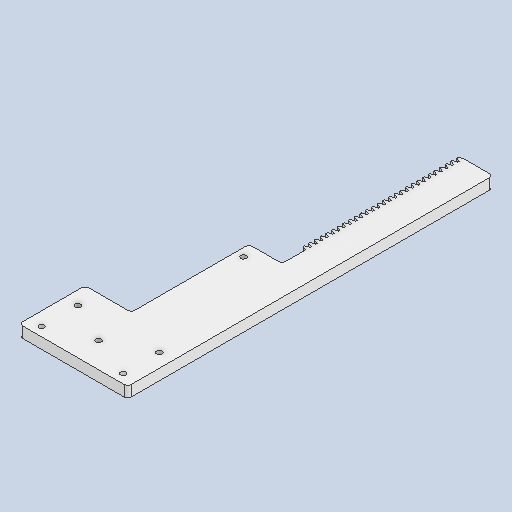
# Autodesk Inventor part: hand-grab-v2-Plate-rack
Saved by Autodesk Inventor 2025.1 (Build 291241000, 241)
## iProperties
Created: 2024-10-12
Part Number: hand-grab-v2-Plate-rack
Material: ABS プラスチック
Document SubType Name: Modeling
Designer: haruy
Density: 1.06 g/cm^3
Appearance: 滑らか - 白
Author: haruy
Autodesk Inventor part; units mm, degrees
ref_plane "YZ Plane" through (0, 0, 0) normal (1, 0, 0) x (0, 1, 0)
ref_plane "XZ Plane" through (0, 0, 0) normal (0, 1, 0) x (-1, 0, 0)
ref_plane "XY Plane" through (0, 0, 0) normal (0, 0, 1) x (1, 0, 0)
derived "hand-grab-v2-Sketch-Base.ipt"
sketch "スケッチ1" plane through (300, 0, 0) normal (1, 0, 0) x (0, 1, 0)
  circle A0 centre (0, 0) radius 122.5
  line L0 (-136.5, 142.5) -> (-132.5, 142.5)
  line L1 (-132.5, 142.5) -> (-132.5, -206.7109)
  line L2 (-132.5, -206.7109) -> (-136.5, -206.7109)
  line L3 (-136.5, -206.7109) -> (-136.5, 142.5)
  line L4 (0, 0) -> (86.6206, 86.6206)
  line L5 (0, 0) -> (0, 122.5)
  line L6 (0, 0) -> (-61.25, 106.0881)
  line L7 (-150.5, 12.2) -> (-198.3, 12.2)
  line L8 (-198.3, 12.2) -> (-198.3, -12.2)
  line L9 (-198.3, -12.2) -> (-150.5, -12.2)
  line L10 (-150.5, -12.2) -> (-150.5, 12.2)
  line L11 (-150.5, 6.5) -> (-147.9, 6.5)
  line L12 (-147.9, 6.5) -> (-147.9, -6.5)
  line L13 (-147.9, -6.5) -> (-150.5, -6.5)
  line L14 (-150.5, -6.5) -> (-150.5, 6.5)
  line L15 (-147.9, 3) -> (-133.5, 3)
  line L16 (-133.5, 3) -> (-133.5, -3)
  line L17 (-133.5, -3) -> (-147.9, -3)
  line L18 (-147.9, -3) -> (-147.9, 3)
  line L19 (-146.5, 70.3296) -> (-150.5, 70.3296)
  line L20 (-150.5, 70.3296) -> (-150.5, -72.1331)
  line L21 (-150.5, -72.1331) -> (-146.5, -72.1331)
  line L22 (-146.5, -72.1331) -> (-146.5, 70.3296)
  line L23 (-136.5, 9) -> (-142.5, 9)
  line L24 (-142.5, 9) -> (-142.5, -9)
  line L25 (-142.5, -9) -> (-136.5, -9)
  line L26 (-136.5, -9) -> (-136.5, 9)
  line L27 (-61.25, 106.0881) -> (-132.5, 106.0881)
  circle A1 centre (-532.5, 0) radius 600
  line L28 (-132.5, 142.5) -> (-7.6064, 142.5)
  arc A2 (86.6206, 86.6206) -> (-7.6064, 142.5) centre (3, 53) ccw
  circle A3 centre (-532.5, 0) radius 400
  circle A4 centre (-332.5, 0) radius 600
sketch "スケッチ2" plane through (0, -300, 0) normal (0, 1, 0) x (-1, 0, 0)
  circle A0 centre (0, 0) radius 122.5
  line L0 (-34, 142.5) -> (-30, 142.5)
  line L1 (-30, 142.5) -> (-30, 106)
  line L2 (-30, 106) -> (-34, 106)
  line L3 (-34, 106) -> (-34, 142.5)
  line L4 (30, 142.5) -> (34, 142.5)
  line L5 (34, 142.5) -> (34, 106)
  line L6 (34, 106) -> (30, 106)
  line L7 (30, 106) -> (30, 142.5)
  circle A1 centre (0, 0) radius 12.5
  line L8 (-30, 142.5) -> (30, 142.5)
  line L9 (-12.5, 103.9737) -> (-12.5, -60) construction
  line L10 (-12.5, -60) -> (-30, -60)
  line L11 (-30, -60) -> (-30, 142.5)
  line L12 (-30, 142.5) -> (-12.5, 142.5)
  line L13 (-12.5, 142.5) -> (-12.5, -60) construction
  line L14 (-30, 20) -> (-12.5, 20) construction
  line L15 (-4.5, 136) -> (4.5, 136) construction
  line L16 (4.5, 136) -> (4.5, 41)
  line L17 (4.5, 41) -> (-4.5, 41) construction
  line L18 (-4.5, 41) -> (-4.5, 136) construction
  line L19 (10, 128.5) -> (-10, 128.5) construction
  line L20 (-10, 128.5) -> (-10, 98.5) construction
  line L21 (-10, 98.5) -> (10, 98.5) construction
  line L22 (10, 98.5) -> (10, 128.5) construction
  line L23 (-12.5, 20) -> (-11.5, 20)
  line L24 (-11.5, 20) -> (-11.5, -60)
  line L25 (-11.5, -60) -> (-12.5, -60)
  line L26 (-12.5, -60) -> (-12.5, 20) construction
  line L27 (-11.5, 20) -> (-13.8, 19.214) construction
  line L28 (-13.8, 19.214) -> (-13.8, 18.429)
  line L29 (-13.8, 18.429) -> (-11.5, 17.643)
  line L30 (-11.5, 17.643) -> (-11.5, 20)
  line L31 (-11.5, 16.8584) -> (-13.8, 16.0724)
  line L32 (-13.8, 15.2874) -> (-11.5, 14.5014)
  line L33 (-13.8, 16.0724) -> (-13.8, 15.2874)
  line L34 (-11.5, 13.7168) -> (-13.8, 12.9308)
  line L35 (-13.8, 12.1458) -> (-11.5, 11.3598)
  line L36 (-13.8, 12.9308) -> (-13.8, 12.1458)
  line L37 (-11.5, 10.5752) -> (-13.8, 9.7892)
  line L38 (-13.8, 9.0042) -> (-11.5, 8.2182)
  line L39 (-13.8, 9.7892) -> (-13.8, 9.0042)
  line L40 (-11.5, 7.4336) -> (-13.8, 6.6476)
  line L41 (-13.8, 5.8626) -> (-11.5, 5.0766)
  line L42 (-13.8, 6.6476) -> (-13.8, 5.8626)
  line L43 (-11.5, 4.292) -> (-13.8, 3.506)
  line L44 (-13.8, 2.721) -> (-11.5, 1.935)
  line L45 (-13.8, 3.506) -> (-13.8, 2.721)
  line L46 (-11.5, 1.1505) -> (-13.8, 0.3645)
  line L47 (-13.8, -0.4205) -> (-11.5, -1.2065)
  line L48 (-13.8, 0.3645) -> (-13.8, -0.4205)
  line L49 (-11.5, -1.9911) -> (-13.8, -2.7771)
  line L50 (-13.8, -3.5621) -> (-11.5, -4.3481)
  line L51 (-13.8, -2.7771) -> (-13.8, -3.5621)
  line L52 (-11.5, -5.1327) -> (-13.8, -5.9187)
  line L53 (-13.8, -6.7037) -> (-11.5, -7.4897)
  line L54 (-13.8, -5.9187) -> (-13.8, -6.7037)
  line L55 (-11.5, -8.2743) -> (-13.8, -9.0603)
  line L56 (-13.8, -9.8453) -> (-11.5, -10.6313)
  line L57 (-13.8, -9.0603) -> (-13.8, -9.8453)
  line L58 (-11.5, -11.4159) -> (-13.8, -12.2019)
  line L59 (-13.8, -12.9869) -> (-11.5, -13.7729)
  line L60 (-13.8, -12.2019) -> (-13.8, -12.9869)
  line L61 (-11.5, -14.5575) -> (-13.8, -15.3435)
  line L62 (-13.8, -16.1285) -> (-11.5, -16.9145)
  line L63 (-13.8, -15.3435) -> (-13.8, -16.1285)
  line L64 (-11.5, -17.6991) -> (-13.8, -18.4851)
  line L65 (-13.8, -19.2701) -> (-11.5, -20.0561)
  line L66 (-13.8, -18.4851) -> (-13.8, -19.2701)
  line L67 (-11.5, -20.8407) -> (-13.8, -21.6267)
  line L68 (-13.8, -22.4117) -> (-11.5, -23.1977)
  line L69 (-13.8, -21.6267) -> (-13.8, -22.4117)
  line L70 (-11.5, -23.9823) -> (-13.8, -24.7683)
  line L71 (-13.8, -25.5533) -> (-11.5, -26.3393)
  line L72 (-13.8, -24.7683) -> (-13.8, -25.5533)
  line L73 (-11.5, -27.1238) -> (-13.8, -27.9099)
  line L74 (-13.8, -28.6949) -> (-11.5, -29.4809)
  line L75 (-13.8, -27.9099) -> (-13.8, -28.6949)
  line L76 (-11.5, -30.2654) -> (-13.8, -31.0514)
  line L77 (-13.8, -31.8364) -> (-11.5, -32.6224)
  line L78 (-13.8, -31.0514) -> (-13.8, -31.8364)
  line L79 (-11.5, -33.407) -> (-13.8, -34.193)
  line L80 (-13.8, -34.978) -> (-11.5, -35.764)
  line L81 (-13.8, -34.193) -> (-13.8, -34.978)
  line L82 (-11.5, -36.5486) -> (-13.8, -37.3346)
  line L83 (-13.8, -38.1196) -> (-11.5, -38.9056)
  line L84 (-13.8, -37.3346) -> (-13.8, -38.1196)
  line L85 (-11.5, -39.6902) -> (-13.8, -40.4762)
  line L86 (-13.8, -41.2612) -> (-11.5, -42.0472)
  line L87 (-13.8, -40.4762) -> (-13.8, -41.2612)
  line L88 (-11.5, -42.8318) -> (-13.8, -43.6178)
  line L89 (-13.8, -44.4028) -> (-11.5, -45.1888)
  line L90 (-13.8, -43.6178) -> (-13.8, -44.4028)
  line L91 (-11.5, -45.9734) -> (-13.8, -46.7594)
  line L92 (-13.8, -47.5444) -> (-11.5, -48.3304)
  line L93 (-13.8, -46.7594) -> (-13.8, -47.5444)
  line L94 (-11.5, -49.115) -> (-13.8, -49.901)
  line L95 (-13.8, -50.686) -> (-11.5, -51.472)
  line L96 (-13.8, -49.901) -> (-13.8, -50.686)
  line L97 (-11.5, -52.2566) -> (-13.8, -53.0426)
  line L98 (-13.8, -53.8276) -> (-11.5, -54.6136)
  line L99 (-13.8, -53.0426) -> (-13.8, -53.8276)
  line L100 (-11.5, -55.3982) -> (-13.8, -56.1842)
  line L101 (-13.8, -56.9692) -> (-11.5, -57.7552)
  line L102 (-13.8, -56.1842) -> (-13.8, -56.9692)
  line L103 (-11.5, -58.5397) -> (-13.8, -59.3258)
  line L104 (-13.8, -60.1108) -> (-11.5, -60.8968)
  line L105 (-13.8, -59.3258) -> (-13.8, -60.1108)
  line L106 (-13.8, 20) -> (-13.8, -60) construction
  line L107 (-13.8, -59.3258) -> (-30, -59.3258)
  line L108 (-13.8, 18.429) -> (-30, 18.429) construction
  line L109 (-13.8, 18.429) -> (-13.8, 142.5)
  line L110 (-34, 137.5) -> (34, 137.5) construction
  line L111 (-34, 117.5) -> (34, 117.5) construction
  line L112 (30, 106) -> (-13.8, 106)
  line L113 (32, -142.5) -> (30, -142.5)
  line L114 (30, -142.5) -> (30, -106)
  line L115 (30, -106) -> (32, -106)
  line L116 (32, -106) -> (32, -142.5)
  line L117 (-32, -106) -> (-30, -106)
  line L118 (-30, -106) -> (-30, -142.5)
  line L119 (-30, -142.5) -> (-32, -142.5)
  line L120 (-32, -142.5) -> (-32, -106)
  line L121 (30, -142.5) -> (-30, -142.5)
  line L122 (30, -142.5) -> (12.5, -142.5)
  line L123 (12.5, -142.5) -> (12.5, 80)
  line L124 (12.5, 80) -> (30, 80)
  line L125 (30, 80) -> (30, -142.5)
  line L126 (-30, -106) -> (12.5, -106)
  line L127 (-4.5, -41) -> (4.5, -41)
  line L128 (4.5, -41) -> (4.5, -136)
  line L129 (4.5, -136) -> (-4.5, -136)
  line L130 (-4.5, -136) -> (-4.5, -41)
  line L131 (-10, -98.5) -> (10, -98.5)
  line L132 (10, -98.5) -> (10, -128.5)
  line L133 (10, -128.5) -> (-10, -128.5)
  line L134 (-10, -128.5) -> (-10, -98.5)
  circle A2 centre (0, 128.5) radius 1.5
  circle A3 centre (0, 48.5) radius 1.5
  line L135 (-32, 202.1278) -> (-17, 202.1278)
  line L136 (-17, 202.1278) -> (-17, -209.3238) construction
  line L137 (-17, -209.3238) -> (-32, -209.3238)
  line L138 (-32, -209.3238) -> (-32, 202.1278) construction
  line L139 (17, 202.1278) -> (32, 202.1278)
  line L140 (32, 202.1278) -> (32, -266.5661) construction
  line L141 (32, -266.5661) -> (17, -266.5661)
  line L142 (17, -266.5661) -> (17, 202.1278) construction
  line L143 (4.5, 41) -> (-13.8, 41)
  line L144 (-30, 30) -> (-12.65, 30) construction
  line L145 (-30, 142.5) -> (-15, 142.5)
  line L146 (-15, 142.5) -> (-15, 106)
  line L147 (-15, 106) -> (-30, 106)
  line L148 (-30, 106) -> (-30, 142.5)
  line L149 (30, 142.5) -> (15, 142.5)
  line L150 (15, 142.5) -> (15, 106)
  line L151 (15, 106) -> (30, 106)
  line L152 (30, 106) -> (30, 142.5)
  line L153 (-13.8, 21.571) -> (-11.5, 20.785)
  line L154 (-11.5, 20.0004) -> (-13.8, 19.2144)
  line L155 (-13.8, 24.713) -> (-11.5, 23.927)
  line L156 (-11.5, 23.1424) -> (-13.8, 22.3564)
  line L157 (-13.8, 27.855) -> (-11.5, 27.069)
  line L158 (-11.5, 26.2844) -> (-13.8, 25.4984)
  line L159 (-13.8, 30.997) -> (-11.5, 30.211)
  line L160 (-11.5, 29.4264) -> (-13.8, 28.6404)
  line L161 (-11.5, 20.0004) -> (-11.5, 27.069)
  line L162 (-13.8, 27.855) -> (-30, 27.855) construction
  circle A4 centre (-22.5, 137.5) radius 1.5
  circle A5 centre (-22.5, 117.5) radius 1.5
  line L163 (0, 0) -> (0, 173.505)
  circle A6 centre (22.5, 137.5) radius 1.5
  circle A7 centre (22.5, 117.5) radius 1.5
  point P0 (21.25, -142.5)
  point P1 (0, 128.5)
  point P2 (-11.5, -4.899)
  point P3 (-11.7508, -4.2624)
  point P4 (-12.2936, -2.2623)
  point P5 (-12.4693, -0.8753)
  point P6 (-12.4732, 0.8179)
  point P7 (-12.3032, 2.2095)
  point P8 (-11.7738, 4.1985)
  point P9 (-11.5, 4.899)
  point P10 (-22.5, 142.5)
  point P11 (4.5, 106)
  point P12 (-13.8, 41)
  dimension "d1" = 3
  dimension "d2" = 3
  dimension "d3" = 4.5
  dimension "d4" = 4.5
  dimension "d5" = 7.5
  dimension "d6" = 80
  dimension "d28" = 3
  dimension "d29" = 3
  dimension "d30" = 7.5
  dimension "d31" = 7.5
  measures "d1" diameter of A2
  measures "d2" diameter of A3
  measures "d3" distance from line of A2.centre L18
  measures "d4" distance from line of A3.centre L18
  measures "d5" distance from line of A2.centre L15
  measures "d6" distance of A3.centre point (0, 128.5)
  measures "d28" diameter of A4
  measures "d29" diameter of A5
  measures "d30" distance from line of A4.centre L11
  measures "d31" distance from line of A5.centre L1
ref_plane "作業平面1" through (0, -300, 0) normal (0, 1, 0) x (-1, 0, 0)
ref_plane "作業平面2" through (300, 0, 0) normal (1, 0, 0) x (0, 1, 0)
extrude "押し出し1" add sketch "スケッチ2" along normal blind 6 contours L7 L112 L150 A0 | A0 L150 L8 L7 | L150 L112 L16 A0 | A0 L163 A2 L8 L150 | L16 L112 L163 A0 | L163 L112 L109 A0 | A0 L109 L8 L163 A2 | L16 L143 L163 A3 L112 | L109 L28 L29 L24 L31 L33 L32 L34 L36 L35 L37 L39 L38 L40 L42 L41 A1 L43 L45 L44 L46 L48 L47 L49 L51 L50 L52 L54 L53 L55 L57 L56 L58 L60 L59 L61 L63 L62 L64 L66 L65 L67 L69 L68 L70 L72 L71 L73 L75 L74 L76 L78 L77 L79 L81 L80 L82 L84 L83 L85 L87 L86 L88 L90 L89 L91 L93 L92 L94 L96 L95 L97 L99 L98 L100 L102 L101 L103 L107 L11 L147 L146 A0 | A0 L146 L8 L109 | L163 A3 L143 L109 L112 | A1 L50 L24 | L146 L147 L1 A0 | A0 L1 L8 L146 | L24 L43 A1 | A1 L47 L24 L49 | L44 L24 L46 A1 | L157 L161 L158 L109 | L155 L161 L156 L109 | L153 L161 L154 L109 | A4 | A5 | A6 | A7
extrude "押し出し2" cut sketch "スケッチ2" along normal through all contours A4 | A5 | A6 | A7
fillet "フィレット1" radius 2 7 edges at (30, -297, 142.5) (-30, -297, 142.5) (-30, -297, 106) (-4.5, -297, 106) (-4.5, -297, 41) (13.8, -297, 41) (30, -297, -59.3258)
sketch "スケッチ4" plane through (-28, -294, 142.5) normal (0, 1, 0) x (1, 0, 0)
  circle A0 centre (28, 94) radius 1.5 projected
  circle A1 centre (28, 14) radius 1.5 projected
  arc A2 (58, 199.8258) -> (56, 201.8258) centre (56, 199.8258) ccw projected
  line L0 (56, 201.8258) -> (41.8, 201.8258) projected
  line L1 (41.8, 201.8258) -> (39.5, 201.0397) projected
  line L2 (39.5, 201.0397) -> (39.5, 200.2552) projected
  line L3 (39.5, 200.2552) -> (41.8, 199.4692) projected
  line L4 (41.8, 199.4692) -> (41.8, 198.6842) projected
  line L5 (41.8, 198.6842) -> (39.5, 197.8982) projected
  line L6 (39.5, 197.8982) -> (39.5, 197.1136) projected
  line L7 (39.5, 197.1136) -> (41.8, 196.3276) projected
  line L8 (41.8, 196.3276) -> (41.8, 195.5426) projected
  line L9 (41.8, 195.5426) -> (39.5, 194.7566) projected
  line L10 (39.5, 194.7566) -> (39.5, 193.972) projected
  line L11 (39.5, 193.972) -> (41.8, 193.186) projected
  line L12 (41.8, 193.186) -> (41.8, 192.401) projected
  line L13 (41.8, 192.401) -> (39.5, 191.615) projected
  line L14 (39.5, 191.615) -> (39.5, 190.8304) projected
  line L15 (39.5, 190.8304) -> (41.8, 190.0444) projected
  line L16 (41.8, 190.0444) -> (41.8, 189.2594) projected
  line L17 (41.8, 189.2594) -> (39.5, 188.4734) projected
  line L18 (39.5, 188.4734) -> (39.5, 187.6888) projected
  line L19 (39.5, 187.6888) -> (41.8, 186.9028) projected
  line L20 (41.8, 186.9028) -> (41.8, 186.1178) projected
  line L21 (41.8, 186.1178) -> (39.5, 185.3318) projected
  line L22 (39.5, 185.3318) -> (39.5, 184.5472) projected
  line L23 (39.5, 184.5472) -> (41.8, 183.7612) projected
  line L24 (41.8, 183.7612) -> (41.8, 182.9762) projected
  line L25 (41.8, 182.9762) -> (39.5, 182.1902) projected
  line L26 (39.5, 182.1902) -> (39.5, 181.4056) projected
  line L27 (39.5, 181.4056) -> (41.8, 180.6196) projected
  line L28 (41.8, 180.6196) -> (41.8, 179.8346) projected
  line L29 (41.8, 179.8346) -> (39.5, 179.0486) projected
  line L30 (39.5, 179.0486) -> (39.5, 178.264) projected
  line L31 (39.5, 178.264) -> (41.8, 177.478) projected
  line L32 (41.8, 177.478) -> (41.8, 176.693) projected
  line L33 (41.8, 176.693) -> (39.5, 175.907) projected
  line L34 (39.5, 175.907) -> (39.5, 175.1224) projected
  line L35 (39.5, 175.1224) -> (41.8, 174.3364) projected
  line L36 (41.8, 174.3364) -> (41.8, 173.5514) projected
  line L37 (41.8, 173.5514) -> (39.5, 172.7654) projected
  line L38 (39.5, 172.7654) -> (39.5, 171.9809) projected
  line L39 (39.5, 171.9809) -> (41.8, 171.1949) projected
  line L40 (41.8, 171.1949) -> (41.8, 170.4099) projected
  line L41 (41.8, 170.4099) -> (39.5, 169.6239) projected
  line L42 (39.5, 169.6239) -> (39.5, 168.8393) projected
  line L43 (39.5, 168.8393) -> (41.8, 168.0533) projected
  line L44 (41.8, 168.0533) -> (41.8, 167.2683) projected
  line L45 (41.8, 167.2683) -> (39.5, 166.4823) projected
  line L46 (39.5, 166.4823) -> (39.5, 165.6977) projected
  line L47 (39.5, 165.6977) -> (41.8, 164.9117) projected
  line L48 (41.8, 164.9117) -> (41.8, 164.1267) projected
  line L49 (41.8, 164.1267) -> (39.5, 163.3407) projected
  line L50 (39.5, 163.3407) -> (39.5, 162.5561) projected
  line L51 (39.5, 162.5561) -> (41.8, 161.7701) projected
  line L52 (41.8, 161.7701) -> (41.8, 160.9851) projected
  line L53 (41.8, 160.9851) -> (39.5, 160.1991) projected
  line L54 (39.5, 160.1991) -> (39.5, 159.4145) projected
  line L55 (39.5, 159.4145) -> (41.8, 158.6285) projected
  line L56 (41.8, 158.6285) -> (41.8, 157.8435) projected
  line L57 (41.8, 157.8435) -> (39.5, 157.0575) projected
  line L58 (39.5, 157.0575) -> (39.5, 156.2729) projected
  line L59 (39.5, 156.2729) -> (41.8, 155.4869) projected
  line L60 (41.8, 155.4869) -> (41.8, 154.7019) projected
  line L61 (41.8, 154.7019) -> (39.5, 153.9159) projected
  line L62 (39.5, 153.9159) -> (39.5, 153.1313) projected
  line L63 (39.5, 153.1313) -> (41.8, 152.3453) projected
  line L64 (41.8, 152.3453) -> (41.8, 151.5603) projected
  line L65 (41.8, 151.5603) -> (39.5, 150.7743) projected
  line L66 (39.5, 150.7743) -> (39.5, 149.9897) projected
  line L67 (39.5, 149.9897) -> (41.8, 149.2037) projected
  line L68 (41.8, 149.2037) -> (41.8, 148.4187) projected
  line L69 (41.8, 148.4187) -> (39.5, 147.6327) projected
  line L70 (39.5, 147.6327) -> (39.5, 146.8481) projected
  line L71 (39.5, 146.8481) -> (41.8, 146.0621) projected
  line L72 (41.8, 146.0621) -> (41.8, 145.2771) projected
  line L73 (41.8, 145.2771) -> (39.5, 144.4911) projected
  line L74 (39.5, 144.4911) -> (39.5, 143.7065) projected
  line L75 (39.5, 143.7065) -> (41.8, 142.9205) projected
  line L76 (41.8, 142.9205) -> (41.8, 142.1355) projected
  line L77 (41.8, 142.1355) -> (39.5, 141.3495) projected
  line L78 (39.5, 141.3495) -> (39.5, 140.565) projected
  line L79 (39.5, 140.565) -> (41.8, 139.779) projected
  line L80 (41.8, 139.779) -> (41.8, 138.994) projected
  line L81 (41.8, 138.994) -> (39.5, 138.208) projected
  line L82 (39.5, 138.208) -> (39.5, 137.4234) projected
  line L83 (39.5, 137.4234) -> (41.8, 136.6374) projected
  line L84 (41.8, 136.6374) -> (41.8, 135.8524) projected
  line L85 (41.8, 135.8524) -> (39.5, 135.0664) projected
  line L86 (39.5, 135.0664) -> (39.5, 134.2818) projected
  line L87 (39.5, 134.2818) -> (41.8, 133.4958) projected
  line L88 (41.8, 133.4958) -> (41.8, 132.7108) projected
  line L89 (41.8, 132.7108) -> (39.5, 131.9248) projected
  line L90 (39.5, 131.9248) -> (39.5, 131.1402) projected
  line L91 (39.5, 131.1402) -> (41.8, 130.3542) projected
  line L92 (41.8, 130.3542) -> (41.8, 129.5692) projected
  line L93 (41.8, 129.5692) -> (39.5, 128.7832) projected
  line L94 (39.5, 128.7832) -> (39.5, 127.9986) projected
  line L95 (39.5, 127.9986) -> (41.8, 127.2126) projected
  line L96 (41.8, 127.2126) -> (41.8, 126.4276) projected
  line L97 (41.8, 126.4276) -> (39.5, 125.6416) projected
  line L98 (39.5, 125.6416) -> (39.5, 124.857) projected
  line L99 (39.5, 124.857) -> (41.8, 124.071) projected
  line L100 (41.8, 124.071) -> (41.8, 123.2856) projected
  line L101 (41.8, 123.2856) -> (39.5, 122.4996) projected
  line L102 (39.5, 122.4996) -> (39.5, 121.715) projected
  line L103 (39.5, 121.715) -> (41.8, 120.929) projected
  line L104 (41.8, 120.929) -> (41.8, 120.1436) projected
  line L105 (41.8, 120.1436) -> (39.5, 119.3576) projected
  line L106 (39.5, 119.3576) -> (39.5, 118.573) projected
  line L107 (39.5, 118.573) -> (41.8, 117.787) projected
  line L108 (41.8, 117.787) -> (41.8, 117.0016) projected
  line L109 (41.8, 117.0016) -> (39.5, 116.2156) projected
  line L110 (39.5, 116.2156) -> (39.5, 115.431) projected
  line L111 (39.5, 115.431) -> (41.8, 114.645) projected
  line L112 (41.8, 114.645) -> (41.8, 103.5) projected
  arc A3 (39.8, 101.5) -> (41.8, 103.5) centre (39.8, 103.5) ccw projected
  line L113 (39.8, 101.5) -> (25.5, 101.5) projected
  arc A4 (25.5, 101.5) -> (23.5, 99.5) centre (25.5, 99.5) ccw projected
  line L114 (23.5, 99.5) -> (23.5, 38.5) projected
  arc A5 (21.5, 36.5) -> (23.5, 38.5) centre (21.5, 38.5) ccw projected
  line L115 (21.5, 36.5) -> (0, 36.5) projected
  arc A6 (0, 36.5) -> (-2, 34.5) centre (0, 34.5) ccw projected
  line L116 (-2, 34.5) -> (-2, 2) projected
  arc A7 (-2, 2) -> (0, 0) centre (0, 2) ccw projected
  line L117 (0, 0) -> (56, 0) projected
  arc A8 (56, 0) -> (58, 2) centre (56, 2) ccw projected
  line L118 (58, 2) -> (58, 199.8258) projected
  point P0 (28, 142.5)
equation "\"d4\" = d3"
equation "\"d31\" = d30"
